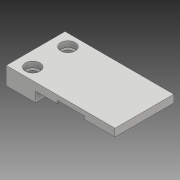
# Autodesk Inventor part: thumb_03 CMC bottom angle sensor holder
Saved by Autodesk Inventor 2017 SP1 (Build 210196100, 196)
## iProperties
Created: 2018-02-11
Part Number: thumb_03 CMC bottom angle sensor holder
Material: Generic
Document SubType Name: Modeling
Designer: JT
Density: 1 g/cm^3
Appearance: Default
Author: JT
Autodesk Inventor part; units mm, degrees
ref_plane "YZ Plane" through (0, 0, 0) normal (1, 0, 0) x (0, 1, 0)
ref_plane "XZ Plane" through (0, 0, 0) normal (0, 1, 0) x (-1, 0, 0)
ref_plane "XY Plane" through (0, 0, 0) normal (0, 0, 1) x (1, 0, 0)
sketch "Sketch1" plane through (0, 0, 0) normal (0, 0, 1) x (1, 0, 0)
  line L0 (0, 0) -> (18.5, 0)
  line L1 (18.5, 0) -> (18.5, 10)
  line L2 (18.5, 10) -> (0, 10)
  line L3 (0, 10) -> (0, 0)
  dimension "d0" = 18.5
  dimension "d1" = 10
  constraints: 8 end point, 2 parallel, 1 horizontal, 1 perpendicular
  measures "d0" distance of L1.end L2.end
  measures "d1" distance of L0.end L1.end
extrude "Extrusion1" add sketch "Sketch1" along normal blind 3
sketch "Sketch2" plane through (0, 0, 0) normal (0, 0, -1) x (-1, 0, 0)
  line L0 (0, 0) -> (-18.5, 0) projected
  line L1 (0, 10) -> (0, 0) projected
  line L2 (-18.5, 10) -> (0, 10) projected
  line L3 (-18.5, 0) -> (-18.5, 10) projected
  line L4 (-5, 10) -> (-5, 0)
  dimension "d4" = 5
  constraints: 2 end point, 2 point on line, 1 perpendicular
  measures "d4" distance between parallel lines of L1 L4
extrude "Extrusion2" cut sketch "Sketch2" against normal blind 1.7 contours L0 L3 L2 L4
sketch "Sketch3" plane through (0, 0, 3) normal (0, 0, 1) x (1, 0, 0)
  point P0 (0, 0)
  point P1 (2.5, 2)
  point P2 (2.5, 8)
  dimension "d7" = 6
  dimension "d8" = 2.5
  dimension "d9" = 2
  constraints: 1 vertical alignment
  measures "d7" distance of point (2.5, 2) point (2.5, 8)
  measures "d8" horizontal distance of point (2.5, 2) point (0, 0)
  measures "d9" vertical distance of point (0, 0) point (2.5, 2)
hole "Hole1" at (2.5, 2, 3) at (2.5, 8, 3) direction (0, 0, -1) diameter 1.5 depth 8 tip angle 118 counterbore diameter 2.5 counterbore depth 1
sketch "Sketch4" plane through (0, 0, 1.7) normal (0, 0, -1) x (-1, 0, 0)
  circle A0 centre (-2.5, 2) radius 0.75 projected
  point P0 (0, 0)
  point P1 (-11, 1)
  dimension "d18" = 8.5
  dimension "d26" = 1
  measures "d18" horizontal distance of A0.centre point (-11, 1)
  measures "d26" vertical distance of point (-11, 1) A0.centre
hole "Hole2" at (11, 1, 1.7) direction (0, 0, 1) diameter 5 depth 0.5
body "Solid1"
